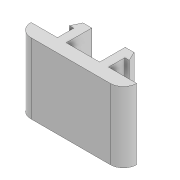
# Autodesk Inventor part: Misumi_Cable_Clip
Saved by Autodesk Inventor 2021 (Build 250183000, 183)
## iProperties
Created: 2021-09-01
Part Number: Misumi_Cable_Clip
Material: Generisch
Document SubType Name: Modeling
Designer: Rama
Density: 1 g/cm^3
Appearance: Vorgabe
Author: Rama
Autodesk Inventor part; units mm, degrees
ref_plane "YZ Plane" through (0, 0, 0) normal (1, 0, 0) x (0, 1, 0)
ref_plane "XZ Plane" through (0, 0, 0) normal (0, 1, 0) x (-1, 0, 0)
ref_plane "XY Plane" through (0, 0, 0) normal (0, 0, 1) x (1, 0, 0)
sketch "Skizze1" plane through (0, 0, 0) normal (0, 1, 0) x (-1, 0, 0)
  line L0 (-6, 0) -> (6, 0)
  arc A0 (-4.5, 1.5) -> (-6, 0) centre (-4.5, 0) ccw
  line L1 (4.5, 1.5) -> (-4.5, 1.5)
  arc A1 (6, 0) -> (4.5, 1.5) centre (4.5, 0) ccw
  line L2 (3.0007, -2.9) -> (3.0007, 0)
  line L3 (2.0007, 0) -> (2.0007, -2.9)
  line L4 (2.0007, -2.9) -> (3.0007, -2.9)
  line L5 (3.0007, -2.9) -> (3.5007, -1.8564)
  line L6 (3.5007, -1.8564) -> (3.0007, -1.8564)
  line L7 (-1.7993, -2.9) -> (-1.7993, 0)
  line L8 (-2.7993, 0) -> (-2.7993, -2.9)
  line L9 (-2.7993, -2.9) -> (-1.7993, -2.9)
  line L10 (-3.2993, -1.8564) -> (-2.7993, -2.9)
  line L11 (-2.7993, -1.8564) -> (-3.2993, -1.8564)
  point P0 (0, 0)
  point P1 (0, 0)
  dimension "d0" = 3
  dimension "d1" = 3
  dimension "d2" = 1
  dimension "d3" = 1
  dimension "d4" = 154.4
  dimension "d5" = 154.4
  dimension "d7" = 0.5
  dimension "d8" = 3.8
  dimension "d9" = 2.9
  dimension "d10" = 9
  dimension "d12" = 5.8
  dimension "d13" = 0.5
  dimension "d14" = 2.9
  dimension "d15" = 4.5
  dimension "d16" = 0
  constraints: 26 end point, 8 point on line, 7 parallel, 4 point on circle, 2 centre point, 2 tangent, 1 coincident
  measures "d0" diameter of A1
  measures "d1" diameter of A0
  measures "d2" distance of L9.start L7.start
  measures "d3" distance of L3.end L4.end
  measures "d4" angle of L8 L10
  measures "d5" angle of L2 L5
  measures "d7" distance of L11.start L10.start
  measures "d8" distance between parallel lines of L7 L3
  measures "d9" distance from line of A1.centre L4
  measures "d10" distance of A1.centre A0.centre
  measures "d12" distance between parallel lines of L2 L8
  measures "d13" distance of L6.start L6.end
  measures "d14" distance of L7.start L7.end
  measures "d15" distance of point (0, 0) A0.centre
  measures "d16" distance from line of point (0, 0) L0
extrude "Extrusion1" add sketch "Skizze1" along normal blind 8
equation "\"d1\" = d0"
equation "\"d3\" = d2"
equation "\"d5\" = d4"
equation "\"d13\" = d7"
equation "\"d15\" = 0.5 * d10"
